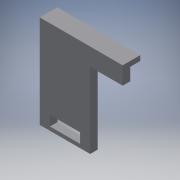
# Autodesk Inventor part: Aligner Helper v3
Saved by Autodesk Inventor 2019 (Build 230136000, 136)
## iProperties
Created: 2021-08-21
Part Number: Aligner Helper v3
Material: Generic
Document SubType Name: Modeling
Designer: Lix
Density: 1 g/cm^3
Appearance: Gold
Author: Lix
Autodesk Inventor part; units mm, degrees
ref_plane "YZ Plane" through (0, 0, 0) normal (1, 0, 0) x (0, 1, 0)
ref_plane "XZ Plane" through (0, 0, 0) normal (0, 1, 0) x (-1, 0, 0)
ref_plane "XY Plane" through (0, 0, 0) normal (0, 0, 1) x (1, 0, 0)
sketch "Sketch1" plane through (0, 0, 0) normal (0, 0, 1) x (1, 0, 0)
  line L0 (-3.1754, 5) -> (-49.0181, 5) projected
  line L1 (-3.1754, 40) -> (-3.1754, 5) projected
  line L2 (-97.8609, 40) -> (-3.1754, 40) projected
  line L3 (-97.8609, 5) -> (-97.8609, 40) projected
  line L4 (-52.0181, 5) -> (-97.8609, 5) projected
  line L5 (-52.0181, 5) -> (-52.0181, 37) projected
  line L6 (-52.0181, 37) -> (-49.0181, 37) projected
  line L7 (-49.0181, 37) -> (-49.0181, 5) projected
  line L8 (-52.0181, 5) -> (-85.0042, 5)
  line L9 (-85.0042, 5) -> (-85.0042, 50)
  line L10 (-85.0042, 50) -> (-52.0181, 50)
  line L11 (-52.0181, 50) -> (-52.0181, 5)
  line L12 (-52.0181, 10.5351) -> (-74.9481, 10.5351) construction
  point P0 (0, 0)
  point P1 (-66.8598, 10.5351)
  dimension "d1" = 45
  dimension "d7" = 45.8427
  dimension "d8" = 22.93
  constraints: 10 end point, 2 parallel, 2 perpendicular, 2 point on line, 1 coincident, 1 horizontal
  measures "d1" distance of L8.end L9.end
  measures "d7" distance between parallel lines of L3 L5
  measures "d8" distance of L12.start L12.end
extrude "Extrusion1" add sketch "Sketch1" along normal blind 3 contours L11 L5 L4 L9 L2 | L2 L9 L10 L11
sketch "Sketch2" plane through (0, 0, 0) normal (0, 0, -1) x (-1, 0, 0)
  line L0 (95.2628, 40) -> (95.2628, 0) projected
  line L1 (5.7735, 40) -> (95.2628, 40) projected
  line L2 (5.7735, 0) -> (5.7735, 40) projected
  line L3 (95.2628, 0) -> (5.7735, 0) projected
  line L4 (52.0181, 5) -> (52.0181, 50) projected
  line L5 (85.0042, 5) -> (52.0181, 5) projected
  line L6 (85.0042, 50) -> (85.0042, 5) projected
  line L7 (52.0181, 50) -> (85.0042, 50) projected
  line L8 (52.0181, 50) -> (85.0042, 50)
  line L9 (85.0042, 50) -> (85.0042, 40)
  line L10 (85.0042, 40) -> (52.0181, 40)
  line L11 (52.0181, 40) -> (52.0181, 50)
  point P0 (0, 0)
  constraints: 8 end point, 2 parallel, 2 point on line, 1 horizontal, 1 perpendicular
extrude "Extrusion2" add sketch "Sketch2" along normal blind 4 contours L1 L4 L7 L6
sketch "Sketch3" plane through (0, 0, 3) normal (0, 0, 1) x (1, 0, 0)
  line L0 (-80.9481, 10.4777) -> (-68.9481, 10.4777)
  line L1 (-68.9481, 10.4777) -> (-68.9481, 6.4777)
  line L2 (-68.9481, 6.4777) -> (-80.9481, 6.4777)
  line L3 (-80.9481, 6.4777) -> (-80.9481, 10.4777)
  line L4 (-80.9481, 10.4777) -> (-68.9481, 6.4777) construction
  line L5 (-68.9481, 10.4777) -> (-80.9481, 6.4777) construction
  circle A0 centre (-74.9481, 8.4777) radius 2 construction
  circle A1 centre (-71.4481, 8.4777) radius 2 construction
  circle A2 centre (-71.7614, 8.4777) radius 2 construction
  line L6 (-52.0181, 5) -> (-52.0181, 50) projected
  point P0 (0, 0)
  point P1 (-71.4481, 8.4777)
  dimension "d9" = 12
  dimension "d10" = 4
  dimension "d11" = 4
  dimension "d12" = 3.5
  dimension "d13" = 3.5
  dimension "d23" = 22.93
  constraints: 12 end point, 3 centre point, 2 coincident, 2 midpoint, 2 parallel, 1 equal radius, 1 horizontal, 1 perpendicular, 1 tangent
  measures "d9" distance of L1.end L2.end
  measures "d10" distance of L0.end L1.end
  measures "d11" diameter of A0
  measures "d12" distance of A1.centre A0.centre
  measures "d13" distance of point (-74.948, 8.478) point (-71.448, 8.478)
  measures "d23" distance from line of L6 A0.centre
extrude "Extrusion3" cut sketch "Sketch3" against normal blind 4
sketch "Sketch5" plane through (0, 0, 3) normal (0, 0, 1) x (1, 0, 0)
  line L0 (-80.9481, 6.4777) -> (-80.9481, 10.4777) projected
  line L1 (-80.9481, 10.4777) -> (-68.9481, 10.4777) projected
  line L2 (-68.9481, 10.4777) -> (-68.9481, 6.4777) projected
  line L3 (-68.9481, 6.4777) -> (-80.9481, 6.4777) projected
  line L4 (-52.0181, 5) -> (-52.0181, 50) projected
  line L5 (-52.0181, 50) -> (-85.0042, 50) projected
  line L6 (-85.0042, 50) -> (-85.0042, 5) projected
  line L7 (-85.0042, 5) -> (-52.0181, 5) projected
  line L8 (-64.9481, 5) -> (-64.9481, 35)
  line L9 (-64.9481, 35) -> (-52.0181, 35)
  point P0 (0, 0)
  dimension "d39" = 30
  dimension "d40" = 4
  constraints: 4 end point, 2 point on line, 1 perpendicular, 1 vertical
  measures "d39" distance of L8.start L8.end
  measures "d40" distance between parallel lines of L8 L2
extrude "Extrusion5" cut sketch "Sketch5" against normal blind 4 contours L7 L8 L9 L4
chamfer "Chamfer1" [suppressed]
sketch "Sketch6" plane through (0, 0, 3) normal (0, 0, 1) x (1, 0, 0)
  line L0 (-64.9481, 35) -> (-52.0181, 35) projected
  line L1 (-52.0181, 35) -> (-52.0181, 50) projected
  line L2 (-52.0181, 50) -> (-85.0042, 50) projected
  line L3 (-85.0042, 50) -> (-85.0042, 5) projected
  line L4 (-85.0042, 5) -> (-64.9481, 5) projected
  line L5 (-64.9481, 5) -> (-64.9481, 35) projected
  line L6 (-80.9481, 6.4777) -> (-80.9481, 10.4777) projected
  line L7 (-80.9481, 10.4777) -> (-68.9481, 10.4777) projected
  line L8 (-68.9481, 10.4777) -> (-68.9481, 6.4777) projected
  line L9 (-68.9481, 6.4777) -> (-80.9481, 6.4777) projected
  line L10 (-52.0181, 35) -> (-52.0181, 50) projected
  line L11 (-85.0042, 50) -> (-52.0181, 50)
  line L12 (-52.0181, 50) -> (-52.0181, 42)
  line L13 (-52.0181, 42) -> (-85.0042, 42)
  line L14 (-85.0042, 42) -> (-85.0042, 50)
  point P0 (0, 0)
  dimension "d44" = 8
  constraints: 8 end point, 2 parallel, 1 horizontal, 1 perpendicular, 1 point on line
  measures "d44" distance of L11.end L12.end
extrude "Extrusion6" cut sketch "Sketch6" against normal blind 12.5 contours L13 L3 L2 L1
sketch "Sketch4" plane through (0, 0, 3) normal (0, 0, 1) x (1, 0, 0)
  line L0 (-80.9481, 6.4777) -> (-80.9481, 10.4777) projected
  line L1 (-80.9481, 10.4777) -> (-68.9481, 10.4777) projected
  line L2 (-68.9481, 10.4777) -> (-68.9481, 6.4777) projected
  line L3 (-68.9481, 6.4777) -> (-80.9481, 6.4777) projected
  line L4 (-52.0181, 5) -> (-52.0181, 50) projected
  line L5 (-52.0181, 50) -> (-85.0042, 50) projected
  line L6 (-85.0042, 50) -> (-85.0042, 5) projected
  line L7 (-85.0042, 5) -> (-52.0181, 5) projected
  line L8 (-81.0042, 47) -> (-56.0181, 47)
  line L9 (-56.0181, 47) -> (-56.0181, 42)
  line L10 (-56.0181, 42) -> (-81.0042, 42)
  line L11 (-81.0042, 42) -> (-81.0042, 47)
  line L12 (-81.0042, 38) -> (-56.0181, 38)
  line L13 (-56.0181, 38) -> (-56.0181, 33)
  line L14 (-56.0181, 33) -> (-81.0042, 33)
  line L15 (-81.0042, 33) -> (-81.0042, 38)
  line L16 (-81.0042, 29) -> (-56.0181, 29)
  line L17 (-56.0181, 29) -> (-56.0181, 24)
  line L18 (-56.0181, 24) -> (-81.0042, 24)
  line L19 (-81.0042, 24) -> (-81.0042, 29)
  line L20 (-81.0042, 20) -> (-56.0181, 20)
  line L21 (-56.0181, 20) -> (-56.0181, 15)
  line L22 (-56.0181, 15) -> (-81.0042, 15)
  line L23 (-81.0042, 15) -> (-81.0042, 20)
  point P0 (0, 0)
  dimension "d24" = 4
  dimension "d25" = 4
  dimension "d26" = 3
  dimension "d27" = 5
  dimension "d30" = 9
  constraints: 32 end point, 2 parallel, 1 horizontal, 1 perpendicular, 1 vertical, 24 other
  measures "d24" distance between parallel lines of L11 L6
  measures "d25" distance between parallel lines of L4 L9
  measures "d26" distance between parallel lines of L5 L8
  measures "d27" distance of L8.end L9.end
  measures "d30" distance of L8.start L12.start
equation "\"d13\" = d12"
equation "\"d25\" = d24"
body "Solid1"
